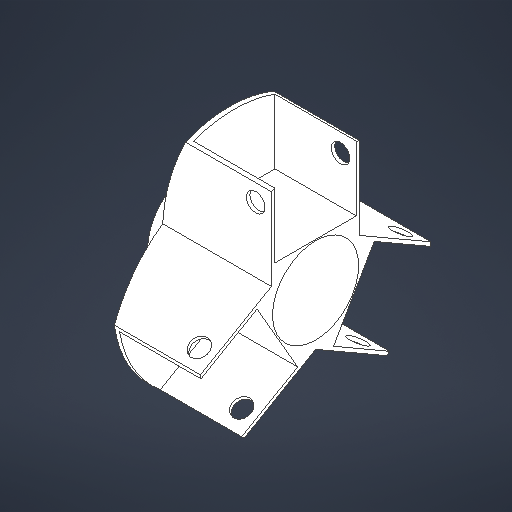
# Autodesk Inventor part: Pieza41
Saved by Autodesk Inventor 2026.2 (Build 302298000, 298)
## iProperties
Created: 2026-01-02
Part Number: Pieza41
Material: Genérico
Document SubType Name: Modeling
Designer: vicho
Density: 1 g/cm^3
Appearance: Valor por defecto
Author: vicho
Autodesk Inventor part; units mm, degrees
ref_plane "YZ Plane" through (0, 0, 0) normal (1, 0, 0) x (0, 1, 0)
ref_plane "XZ Plane" through (0, 0, 0) normal (0, 1, 0) x (-1, 0, 0)
ref_plane "XY Plane" through (0, 0, 0) normal (0, 0, 1) x (1, 0, 0)
sketch "Boceto1" plane through (0, 0, 0) normal (0, 1, 0) x (-1, 0, 0)
  line L0 (116.8368, 0) -> (-138.9188, 0) construction
  line L1 (0, 201.6217) -> (0, -202.3506) construction
  line L2 (-16.9655, 0) -> (-16.9655, 50)
  line L3 (-16.9655, 50) -> (20.0345, 50)
  spline S0 degree 2 poles (20.0345, 50) (29.4829, 31.811) (30.3202, 17.0589) knots 0 0 0 1 1 1
  line L4 (30.3202, 17.0589) -> (30.3202, 0)
  line L5 (30.3202, 0) -> (-16.9655, 0)
  point P0 (0, 0)
  point P1 (27.7444, 31.3016)
  dimension "d0" = 50
  dimension "d1" = 37
  dimension "d2" = 30.3202
  dimension "d3" = 47.2856
  dimension "d4" = 86.5167
  dimension "d5" = 32.9412
  dimension "d6" = 2.5758
  dimension "d7" = 18.6984
  dimension "d8" = 151.6217
  dimension "d9" = 252.3506
  dimension "d10" = 169.239
  constraints: 12 end point, 4 point on line, 2 horizontal, 2 perpendicular, 2 vertical, 3 other
  measures "d0" distance of L2.start L2.end
  measures "d1" distance of L2.end L3.end
  measures "d2" distance between parallel lines of L1 L4
  measures "d3" distance between parallel lines of L4 L2
  measures "d4" distance from line of L0.start L4
  measures "d5" distance from line of L4.start L3
  measures "d6" distance from line of point (27.744, 31.302) L4
  measures "d7" distance from line of point (27.744, 31.302) L3
  measures "d8" distance from line of L1.start L3
  measures "d9" distance from line of L1.end L3
  measures "d10" distance from line of L0.end L4
revolve "Revolución1" add sketch "Boceto1" angle 360 about axis through (-116.8368, 0, 0) along (1, 0, 0)
sketch "Boceto2" plane through (-30.3202, 0, 0) normal (-1, 0, 0) x (0, 0, 1)
  circle A0 centre (0, 0) radius 17.0589 projected
  circle A1 centre (0, 0) radius 21
  point P0 (17.0589, 0)
  dimension "d12" = 42
  constraints: 1 centre point, 1 coincident, 1 horizontal alignment
  measures "d12" diameter of A1
extrude "Extrusión1" add sketch "Boceto2" along normal mid plane 8 contours A0 | A1
sketch "Boceto3" plane through (-34.3202, 0, 0) normal (-1, 0, 0) x (0, 0, 1)
  circle A0 centre (0, 0) radius 18.5
  dimension "d15" = 37
  constraints: 1 centre point, 1 coincident
  measures "d15" diameter of A0
extrude "Extrusión2" cut sketch "Boceto3" against normal blind 60
sketch "Boceto4" plane through (-34.3202, 0, 0) normal (-1, 0, 0) x (0, 0, 1)
  circle A0 centre (0, 0) radius 50 projected
  line L0 (-19, 46.2493) -> (-19, 8.9443)
  circle A1 centre (0, 0) radius 21 projected
  line L1 (19, 46.2493) -> (19, 8.9443)
  line L2 (0, 54.3807) -> (0, -24.3097) construction
  line L3 (-65.0318, 0) -> (77.048, 0) construction
  circle A2 centre (0, 0) radius 50 construction
  circle A3 centre (0, 0) radius 21 construction
  line L4 (-30.5531, -39.5791) -> (1.754, -20.9266)
  line L5 (-49.5531, -6.6702) -> (-17.246, 11.9823)
  circle A4 centre (0, 0) radius 21 construction
  circle A5 centre (0, 0) radius 50 construction
  line L6 (49.5531, -6.6702) -> (17.246, 11.9823)
  line L7 (30.5531, -39.5791) -> (-1.754, -20.9266)
  circle A6 centre (0, 0) radius 21 construction
  circle A7 centre (0, 0) radius 50 construction
  point P0 (19, 10.9697)
  point P1 (-19, 10.9697)
  point P2 (0, -21.9393)
  dimension "d18" = 38
  dimension "d21" = 360
  constraints: 16 end point, 6 centre point, 4 coincident, 4 point on circle, 2 concentric, 2 point on line, 2 vertical, 32 other
  measures "d18" distance between parallel lines of L1 L0
extrude "Extrusión3" cut sketch "Boceto4" against normal blind 60 contours A0 L6 L1 | L0 L5 A0 | A0 L4 L7
sketch "Boceto5" plane through (-29.8214, -21.9393, 0) normal (0, -0.866, -0.5) x (1, 0, 0)
  line L0 (0, 35.9798) -> (0, -55.1659) construction
  line L1 (-10.6314, 0) -> (61.9402, 0) construction
  circle A0 centre (40, 28) radius 4
  point P0 (29.8214, -10.9697)
  point P1 (0, 0)
  dimension "d25" = 40
  dimension "d26" = 28
  dimension "d27" = 8
  constraints: 4 end point, 2 point on line, 1 centre point, 1 coincident, 1 horizontal, 1 vertical
  measures "d25" distance from line of point (40, 28) L0
  measures "d26" distance from line of point (40, 28) L1
  measures "d27" diameter of A0
extrude "Extrusión4" cut sketch "Boceto5" against normal blind 60
pattern_circular "Patrón circular1" count 3 over 360 about axis through (-34.3202, 0, 0) along (1, 0, 0) of "Extrusión4"
sketch "Boceto6" plane through (16.9655, 10.9697, 19) normal (1, 0, 0) x (0, 0, -1)
  line L0 (36.5, 8.0303) -> (1.5, 8.0303)
  line L1 (1.5, 8.0303) -> (1.5, 43.8507)
  line L2 (1.5, 43.8507) -> (36.5, 43.8507)
  line L3 (36.5, 43.8507) -> (36.5, 8.0303)
  line L4 (19, 66.8345) -> (19, -59.037) construction
  line L5 (-55.9645, -10.9697) -> (107.3868, -10.9697) construction
  line L6 (-19.7258, -53.5353) -> (-37.2258, -23.2244)
  line L7 (11.2955, -35.6251) -> (-19.7258, -53.5353)
  line L8 (-37.2258, -23.2244) -> (-6.2045, -5.3142)
  line L9 (-6.2045, -5.3142) -> (11.2955, -35.6251)
  line L10 (75.2258, -23.2244) -> (57.7258, -53.5353)
  line L11 (44.2045, -5.3142) -> (75.2258, -23.2244)
  line L12 (57.7258, -53.5353) -> (26.7045, -35.6251)
  line L13 (26.7045, -35.6251) -> (44.2045, -5.3142)
  point P0 (19, -10.9697)
  point P1 (25.7111, -10.9697)
  dimension "d33" = 35
  dimension "d34" = 35.8203
  dimension "d35" = 19
  dimension "d38" = 360
  constraints: 28 end point, 3 perpendicular, 2 horizontal, 2 vertical, 1 midpoint, 27 other
  measures "d33" distance between parallel lines of L3 L1
  measures "d34" distance between parallel lines of L0 L2
  measures "d35" distance from line of point (19, -10.97) L0
extrude "Extrusión5" cut sketch "Boceto6" against normal blind 35
